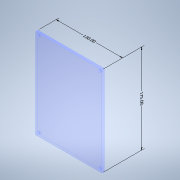
# Autodesk Inventor part: basePlate
Saved by Autodesk Inventor 2022.6 (Build 266554010, 554A)
## iProperties
Created: 2025-03-20
Part Number: basePlate
Material: Generic
Document SubType Name: Modeling
Designer: khinm
Density: 1 g/cm^3
Appearance: Clear - Blue
Author: khinm
Autodesk Inventor part; units mm, degrees
ref_plane "XY Plane" through (0, 0, 0) normal (0, 0, 1) x (1, 0, 0)
sketch "Sketch2" plane through (0, 0, 0) normal (0, 0, 1) x (1, 0, 0)
  line L0 (0, 175) -> (130, 175)
  line L1 (130, 175) -> (130, 0)
  line L2 (130, 0) -> (0, 0)
  line L3 (0, 0) -> (0, 175)
  dimension "d2" = 175
  dimension "d3" = 130
  constraints: 8 end point, 2 parallel, 1 coincident, 1 horizontal, 1 perpendicular
  measures "d2" distance of L0.end L1.end
  measures "d3" distance of L1.end L2.end
extrude "Extrusion1" add sketch "Sketch2" along normal blind 5
sketch "Sketch3" plane through (0, 0, 5) normal (0, 0, 1) x (1, 0, 0)
  line L0 (130, 175) -> (0, 175) projected
  line L1 (0, 0) -> (130, 0) projected
  line L2 (0, 175) -> (0, 0) projected
  line L3 (130, 0) -> (130, 175) projected
  point P0 (5, 170)
  dimension "d8" = 5
  dimension "d9" = 5
  measures "d8" distance from line of L0 point (5, 170)
  measures "d9" distance from line of L2 point (5, 170)
hole "Hole1" at (5, 170, 5) direction (0, 0, -1) diameter 5 depth 5
ref_plane "Work Plane1" through (65, 0, 0) normal (1, 0, 0) x (0, 1, 0)
mirror "Mirror1" about plane through (65, 0, 0) normal (1, 0, 0) of "Hole1"
ref_plane "Work Plane2" through (0, 87.5, 0) normal (0, 1, 0) x (-1, 0, 0)
mirror "Mirror2" about plane through (0, 87.5, 0) normal (0, 1, 0) of "Hole1", "Mirror1"
body "Solid1"
